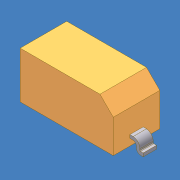
# Autodesk Inventor part: Cap1 SMT
Saved by Autodesk Inventor 2012 (Build 160160000, 160)
## iProperties
Shininess: 64.0
Length Units: 11269
Angle Units: 11279
Time Units: 11290
Mass Units: 11283
Length Display Precision: 3
Angle Display Precision: 2
Compacted: True
Part Number: Cap1 SMT
Document SubType Name: Modeling
Created: 2007-08-26
Material: Delrin, White
Designer: uidk0133
Density: 1.42 g/cm^3
Mass: 0.015038 g
Surface Area: 0.316667 cm^2
Volume: 0.0105902 cm^3
Density: 0.0
Volumn: 0.0
Area: 0.0
PropertySet Name: Model Information
Control State: 0
Master: False
Checked Out: False
Author: uidk0133
Autodesk Inventor part; units mm, degrees
ref_plane "YZ Plane" through (0, 0, 0) normal (1, 0, 0) x (0, 1, 0)
ref_plane "XZ Plane" through (0, 0, 0) normal (0, 1, 0) x (-1, 0, 0)
sketch "Sketch1" plane through (0, 0, 0) normal (0, 0, 1) x (1, 0, 0)
  line L0 (-1.75, 0.875) -> (1.75, 0.875)
  line L1 (1.75, 0.875) -> (1.75, -0.875)
  line L2 (1.75, -0.875) -> (-1.75, -0.875)
  line L3 (-1.75, -0.875) -> (-1.75, 0.875)
  line L4 (0, 0) -> (0, 0.875) construction
  line L5 (0, 0) -> (-1.75, 0) construction
  line L6 (0, 0) -> (1.75, 0) construction
  line L7 (0, 0) -> (0, -0.875) construction
  dimension "d0" = 1.75
  dimension "d1" = 3.5
  constraints: 16 end point, 4 midpoint, 2 collinear, 2 parallel, 1 coincident, 1 horizontal, 1 perpendicular, 2 other
  measures "d0" distance of L0.end L1.end
  measures "d1" distance of L0.start L0.end
extrude "Extrusion1" add sketch "Sketch1" along normal mid plane 1.75
chamfer "Chamfer1" distance 0.5 angle 45 1 edges at (1.75, 0, 0.875)
sketch "Sketch2" plane through (1.75, -0.875, -0.875) normal (1, 0, 0) x (0, 0, -1)
  line L0 (-1.25, 0) -> (0, 0) projected
  line L1 (0, 0) -> (0, 1.75) projected
  line L2 (-1.25, 1.75) -> (0, 1.75) projected
  line L3 (-0.375, 1.125) -> (-0.25, 1.125)
  line L4 (-0.25, 1.125) -> (-0.25, 0.625)
  line L5 (-0.25, 0.625) -> (-0.375, 0.625)
  line L6 (-0.375, 0.625) -> (-0.375, 1.125)
  line L7 (-0.3125, 1.125) -> (-0.3125, 1.75) construction
  line L8 (-0.3125, 0.625) -> (-0.3125, 0) construction
  dimension "d6" = 0.25
  dimension "d7" = 0.5
  dimension "d8" = 0.125
  constraints: 12 end point, 3 equal length, 2 midpoint, 2 perpendicular, 2 point on line, 1 collinear, 1 horizontal
  measures "d6" distance between parallel lines of L4 L1
  measures "d7" distance of L3.end L4.end
  measures "d8" distance of L3.start L3.end
ref_plane "Work Plane2" through (1.75, -0.25, -0.625) normal (0, 1, 0) x (0, 0, 1)
sketch "Sketch4" plane through (1.75, -0.25, -0.625) normal (0, 1, 0) x (0, 0, 1)
  line L0 (0, 0) -> (0.125, 0) projected
  line L1 (0, 0) -> (0, 0.1)
  line L2 (-0.15, 0.25) -> (-0.2, 0.25)
  line L3 (-0.35, 0.4) -> (-0.35, 0.5)
  arc A0 (0, 0.1) -> (-0.15, 0.25) centre (-0.15, 0.1) ccw
  arc A1 (-0.35, 0.4) -> (-0.2, 0.25) centre (-0.2, 0.4) ccw
  point P0 (0, 0.25)
  point P1 (-0.35, 0.25)
  dimension "d11" = 0.25
  dimension "d12" = 0.25
  dimension "d13" = 0.35
  dimension "d14" = 0.15
  constraints: 6 end point, 4 point on circle, 4 point on line, 4 tangent, 2 centre point, 2 perpendicular, 1 equal radius, 1 parallel
  measures "d11" distance of point (-0.35, 0.25) L3.end
  measures "d12" distance of L0.start point (0, 0.25)
  measures "d13" distance of point (0, 0.25) point (-0.35, 0.25)
  measures "d14" radius of A0
sweep "Sweep1" add profiles "Sketch2" path "Sketch4"
mirror "Mirror1" about plane through (0, 0, 0) normal (1, 0, 0) of "Sweep1"
body "Solid1"
